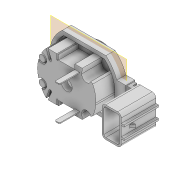
# Autodesk Inventor part: Holder750
Saved by Autodesk Inventor 2021 (Build 250183000, 183)
## iProperties
Created: 2025-07-03
Part Number: Holder750
Material: Generic
Document SubType Name: Modeling
Designer: Owner
Density: 1 g/cm^3
Appearance: Default
Author: Owner
Autodesk Inventor part; units mm, degrees
ref_plane "YZ Plane" through (0, 0, 0) normal (1, 0, 0) x (0, 1, 0)
ref_plane "XZ Plane" through (0, 0, 0) normal (0, 1, 0) x (-1, 0, 0)
ref_plane "XY Plane" through (0, 0, 0) normal (0, 0, 1) x (1, 0, 0)
sketch "Sketch1" plane through (0, 0, 0) normal (0, 0, 1) x (1, 0, 0)
  line L0 (-12, -15.2) -> (12, -15.2)
  line L1 (12, 15.2) -> (-12, 15.2)
  line L2 (-19, -15.2) -> (19, 15.2) construction
  line L3 (19, -15.2) -> (-19, 15.2) construction
  arc A0 (-12, 15.2) -> (-19, 0) centre (1.0029, 0) ccw
  arc A1 (-19, 0) -> (-12, -15.2) centre (1.0029, 0) ccw
  line L4 (-19, -15.2) -> (19, 15.2) construction
  arc A2 (19, 0) -> (12, 15.2) centre (-1.0029, 0) ccw
  arc A3 (12, -15.2) -> (19, 0) centre (-1.0029, 0) ccw
  point P0 (0, 0)
  dimension "d0" = 38
  dimension "d1" = 30.4
  dimension "d2" = 7
  constraints: 10 end point, 8 point on circle, 4 centre point, 2 midpoint, 1 horizontal, 1 parallel
  measures "d0" distance of L3.end L2.end
  measures "d1" distance of L2.end L3.start
  measures "d2" distance of L1.end L3.end
extrude "Extrusion1" add sketch "Sketch1" along normal blind 5
sketch "Sketch2" plane through (0, 0, 5) normal (0, 0, 1) x (1, 0, 0)
  arc A0 (12, -15.2) -> (12, 15.2) centre (-1.0029, 0) ccw projected
  line L0 (12, 15.2) -> (-12, 15.2) projected
  arc A1 (-12, 15.2) -> (-12, -15.2) centre (1.0029, 0) ccw projected
  line L1 (-12, -15.2) -> (12, -15.2) projected
  arc A2 (11.239, -13.2) -> (11.239, 13.2) centre (-1.0029, 0) ccw
  line L2 (11.239, -13.2) -> (-11.239, -13.2)
  arc A3 (-11.239, 13.2) -> (-11.239, -13.2) centre (1.0029, 0) ccw
  line L3 (-11.239, 13.2) -> (11.239, 13.2)
  point P0 (0, 0)
  dimension "d5" = 2
  constraints: 4 end point, 4 point on circle, 2 centre point, 3 other
  measures "d5" radial gap between concentric circles of A0 A2
extrude "Extrusion2" cut sketch "Sketch2" against normal blind 5 contours L2 A3 L3 A2
ref_plane "Work Plane1" through (0, 0, 2.5) normal (0, 0, 1) x (1, 0, 0)
sketch "Sketch3" plane through (0, 0, 2.5) normal (0, 0, 1) x (1, 0, 0)
  arc A0 (11.239, -13.2) -> (11.239, 13.2) centre (-1.0029, 0) ccw projected
  line L0 (11.239, 13.2) -> (-11.239, 13.2) projected
  arc A1 (-11.239, 13.2) -> (-11.239, -13.2) centre (1.0029, 0) ccw projected
  line L1 (-11.239, -13.2) -> (11.239, -13.2) projected
  arc A2 (12, -15.2) -> (12, 15.2) centre (-1.0029, 0) ccw projected
  line L2 (-12, -15.2) -> (12, -15.2) projected
  arc A3 (-12, 15.2) -> (-12, -15.2) centre (1.0029, 0) ccw projected
  line L3 (12, 15.2) -> (-12, 15.2) projected
  line L4 (-5.3682, -1.8242) -> (5.3682, -1.8242)
  arc A4 (5.3682, -1.8242) -> (5.3682, 1.8242) centre (-1.0029, 0) ccw
  line L5 (5.3682, 1.8242) -> (-5.3682, 1.8242)
  arc A5 (-5.3682, 1.8242) -> (-5.3682, -1.8242) centre (1.0029, 0) ccw
  point P0 (0, 0)
  constraints: 4 end point, 4 point on circle, 2 centre point, 3 other
extrude "Extrusion3" add sketch "Sketch3" against normal blind 1 contours L1 A1 L0 A0
sketch "Sketch4" plane through (0, 0, 1.5) normal (0, 0, -1) x (-1, 0, 0)
  circle A0 centre (0, 0) radius 11.25
  dimension "d10" = 22.5
  constraints: 1 centre point, 1 coincident
  measures "d10" diameter of A0
extrude "Extrusion4" add sketch "Sketch4" along normal blind 6
sketch "Sketch5" plane through (0, 0, 2.5) normal (0, 0, 1) x (1, 0, 0)
  arc A0 (11.239, -13.2) -> (11.239, 13.2) centre (-1.0029, 0) ccw projected
  line L0 (11.239, -13.2) -> (-11.239, -13.2) projected
  arc A1 (-11.239, 13.2) -> (-11.239, -13.2) centre (1.0029, 0) ccw projected
  line L1 (-11.239, 13.2) -> (11.239, 13.2) projected
  arc A2 (12, -15.2) -> (12, 15.2) centre (-1.0029, 0) ccw projected
  line L2 (12, 15.2) -> (-12, 15.2) projected
  arc A3 (-12, 15.2) -> (-12, -15.2) centre (1.0029, 0) ccw projected
  line L3 (-12, -15.2) -> (12, -15.2) projected
  arc A4 (5.3351, -1.7805) -> (5.3351, 1.7805) centre (-1.0029, 0) ccw
  line L4 (5.3351, -1.7805) -> (-5.3351, -1.7805)
  arc A5 (-5.3351, 1.7805) -> (-5.3351, -1.7805) centre (1.0029, 0) ccw
  line L5 (-5.3351, 1.7805) -> (5.3351, 1.7805)
  point P0 (0, 0)
  constraints: 4 end point, 4 point on circle, 2 centre point, 3 other
extrude "Extrusion5" add sketch "Sketch5" along normal blind 1 contours L0 A1 L1 A0
sketch "Sketch6" plane through (0, 0, 3.5) normal (0, 0, 1) x (1, 0, 0)
  arc A0 (11.239, -13.2) -> (11.239, 13.2) centre (-1.0029, 0) ccw projected
  line L0 (11.239, -13.2) -> (-11.239, -13.2) projected
  arc A1 (-11.239, 13.2) -> (-11.239, -13.2) centre (1.0029, 0) ccw projected
  line L1 (-11.239, 13.2) -> (11.239, 13.2) projected
  arc A2 (12, -15.2) -> (12, 15.2) centre (-1.0029, 0) ccw projected
  line L2 (12, 15.2) -> (-12, 15.2) projected
  arc A3 (-12, 15.2) -> (-12, -15.2) centre (1.0029, 0) ccw projected
  line L3 (-12, -15.2) -> (12, -15.2) projected
  line L4 (4.5, -14.8235) -> (-4.5, -14.8235)
  line L5 (-4.5, -9.5765) -> (4.5, -9.5765)
  line L6 (4.5, -9.5765) -> (4.5, -12.2)
  line L7 (4.5, -14.8235) -> (-4.5, -9.5765) construction
  line L8 (-4.5, -14.8235) -> (4.5, -9.5765) construction
  line L9 (-4.5, -12.2) -> (-4.5, -9.5765)
  line L10 (4.5, -12.2) -> (8.5, -12.2)
  circle A4 centre (0, 0) radius 3
  line L11 (4.5, -12.2) -> (8.5, -12.2)
  line L12 (15.9256, -1.5884) -> (15.991, -0.5538)
  arc A5 (11.239, -13.2) -> (11.239, 13.2) centre (-1.0029, 0) ccw projected
  arc A6 (13.2862, -8.3182) -> (8.2507, -9.4329) centre (10.8402, -9.1996) ccw
  arc A7 (14.2307, -7.5522) -> (14.2307, 7.5522) centre (-1.0029, 0) ccw
  line L13 (14.2307, -7.5522) -> (13.2862, -8.3182)
  line L14 (8.5, -12.2) -> (8.2507, -9.4329)
  line L15 (-4.8613, -12.2) -> (-4.8613, -9.2)
  line L16 (-4.8613, -9.2) -> (-5.3613, -9.2)
  line L17 (-5.3613, -9.2) -> (-5.3613, -12.2)
  line L18 (-10.2634, -12.2) -> (-5.3613, -12.2)
  line L19 (-4.8613, -12.2) -> (-4.5, -12.2)
  line L20 (-10.2634, -12.2) -> (-5.8402, -12.2) construction
  arc A8 (-8.3701, -7.8223) -> (-9.7725, -7.2951) centre (-9.0585, -7.5245) ccw
  line L21 (-8.3701, -7.8223) -> (-10.2634, -12.2)
  line L22 (-9.7725, -7.2951) -> (-11.2245, -11.8148)
  line L23 (-16, 0) -> (-15.9992, -0.1657)
  circle A9 centre (-13.4708, -5.9877) radius 1.75
  arc A10 (-13.7382, -8.4734) -> (-11.2245, -11.8148) centre (1.0029, 0) ccw
  line L24 (17, 0) -> (-17, 0)
  line L25 (-4.5, 9.5765) -> (4.5, 9.5765)
  line L26 (4.5, 9.5765) -> (4.5, 12.2)
  line L27 (4.5, 14.8235) -> (-4.5, 9.5765) construction
  line L28 (-4.5, 14.8235) -> (4.5, 9.5765) construction
  line L29 (-4.5, 12.2) -> (-4.5, 9.5765)
  line L30 (4.5, 12.2) -> (8.5, 12.2)
  line L31 (4.5, 12.2) -> (8.5, 12.2)
  arc A11 (8.2507, 9.4329) -> (13.2862, 8.3182) centre (10.8402, 9.1996) ccw
  line L32 (14.2307, 7.5522) -> (13.2862, 8.3182)
  line L33 (8.5, 12.2) -> (8.2507, 9.4329)
  line L34 (-4.8613, 12.2) -> (-4.8613, 9.2)
  line L35 (-4.8613, 9.2) -> (-5.3613, 9.2)
  line L36 (-5.3613, 9.2) -> (-5.3613, 12.2)
  line L37 (-10.2634, 12.2) -> (-5.3613, 12.2)
  line L38 (-4.8613, 12.2) -> (-4.5, 12.2)
  line L39 (-10.2634, 12.2) -> (-5.8402, 12.2) construction
  arc A12 (-9.7725, 7.2951) -> (-8.3701, 7.8223) centre (-9.0585, 7.5245) ccw
  line L40 (-8.3701, 7.8223) -> (-10.2634, 12.2)
  line L41 (-9.7725, 7.2951) -> (-11.2245, 11.8148)
  circle A13 centre (-13.4708, 5.9877) radius 1.75
  arc A14 (-11.2245, 11.8148) -> (-13.7382, 8.4734) centre (1.0029, 0) ccw
  line L42 (8.5, 12.2) -> (4.5, 12.2)
  line L43 (-4.5, 12.2) -> (-4.8613, 12.2)
  line L44 (-5.3613, 12.2) -> (-10.2634, 12.2)
  arc A15 (-11.2245, 11.8148) -> (-13.7382, 8.4734) centre (1.0029, 0) ccw
  arc A16 (-15.4161, 4.4175) -> (-15.4161, -4.4175) centre (1.0029, 0) ccw
  circle A17 centre (-13.4708, -5.9877) radius 2.5
  circle A18 centre (-13.4708, 5.9877) radius 2.5
  point P0 (-15.1194, -5.4008)
  point P1 (-14.2229, -7.5679)
  point P2 (15.9256, 1.5884)
  point P3 (-15.1194, 5.4008)
  point P4 (-14.2229, 7.5679)
  dimension "d16" = 9
  dimension "d17" = 6
  dimension "d18" = 4
  dimension "d19" = 6.2
  dimension "d20" = 5.2
  dimension "d21" = 0.5
  dimension "d24" = 1.5
  dimension "d27" = 3.5
  dimension "d28" = 5
  dimension "d29" = 5
  dimension "d32" = 3
  constraints: 82 end point, 32 point on circle, 25 symmetric about line, 14 centre point, 3 coincident, 3 parallel, 3 tangent, 2 horizontal, 1 perpendicular, 4 other
  measures "d16" distance of L5.start L5.end
  measures "d17" diameter of A4
  measures "d18" distance of L10.end L6.end
  measures "d19" distance of L13.start L12.start
  measures "d20" diameter of A6
  measures "d21" distance of L16.end L15.end
  measures "d24" diameter of A8
  measures "d27" diameter of A9
  measures "d28" diameter of A17
  measures "d29" diameter of A18
  measures "d32" distance of L16.end L17.end
extrude "Extrusion6" add sketch "Sketch6" along normal blind 11 contours L24 A4 A16 A18 A14 L41 A12 L40 L37 L36 L35 L34 L38 L29 L25 L26 L30 L33 A11 L32 A7 | A7 L12 L13 A6 L14 L10 L6 L5 L9 L19 L15 L16 L17 L18 L21 A8 L22 A10 A17 A16 L23 L24 A4 | A9 | A13
sketch "Sketch7" plane through (0, 0, 14.5) normal (0, 0, 1) x (1, 0, 0)
  line L0 (-4.5, -9.5765) -> (4.5, -9.5765) projected
  line L1 (4.5, -9.5765) -> (7, -9.5765)
  line L2 (7, -9.5765) -> (7, -9.0765)
  line L3 (7, -9.0765) -> (4.5, -9.0765)
  line L4 (4.5, -9.0765) -> (4.5, -9.5765)
  arc A0 (11.239, -13.2) -> (11.239, 13.2) centre (-1.0029, 0) ccw projected
  line L5 (4.5, 9.5765) -> (7, 9.5765)
  line L6 (7, 9.5765) -> (7, 9.0765)
  line L7 (7, 9.0765) -> (4.5, 9.0765)
  line L8 (4.5, 9.0765) -> (4.5, 9.5765)
  point P0 (0, 0)
  dimension "d33" = 2.5
  dimension "d34" = 0.5
  constraints: 16 end point, 2 parallel, 1 horizontal, 1 perpendicular
  measures "d33" distance of L3.end L2.end
  measures "d34" distance of L2.end L1.end
extrude "Extrusion7" add sketch "Sketch7" along normal blind 11
chamfer "Chamfer1" distance 0.5 angle 45 4 edges at (4.5, -9.3265, 25.5) (7, -9.3265, 25.5) (7, 9.3265, 25.5) (4.5, 9.3265, 25.5)
sketch "Sketch8" plane through (0, 0, 5) normal (0, 0, 1) x (1, 0, 0)
  arc A0 (12, -15.2) -> (12, 15.2) centre (-1.0029, 0) ccw projected
  line L0 (19, 6.5) -> (17.9144, 6.5)
  line L1 (19, -6.5) -> (17.9144, -6.5)
  line L2 (17.9144, -6.5) -> (22.9144, -6.5)
  line L3 (22.9144, -6.5) -> (22.9144, 6.5)
  line L4 (22.9144, 6.5) -> (17.9144, 6.5)
  point P0 (0, 0)
  point P1 (19, 0)
  dimension "d40" = 6.5
  dimension "d41" = 6.5
  dimension "d42" = 5
  constraints: 10 end point, 3 point on circle, 2 perpendicular, 1 horizontal, 1 parallel
  measures "d40" distance of point (19, 0) L1.start
  measures "d41" distance of point (19, 0) L0.start
  measures "d42" distance of L1.end L2.end
extrude "Extrusion8" add sketch "Sketch8" against normal blind 5
sketch "Sketch9" plane through (22.9144, -6.5, 5) normal (1, 0, 0) x (0, 0, -1)
  line L0 (0, 0) -> (0, 13) projected
  line L1 (0, 0) -> (5, 0) projected
  line L2 (5, 13) -> (5, 0) projected
  line L3 (0, 13) -> (5, 13) projected
  line L4 (4.5, 0.5) -> (0.5, 0.5)
  line L5 (0.5, 0.5) -> (0.5, 12.5)
  line L6 (0.5, 12.5) -> (4.5, 12.5)
  line L7 (4.5, 12.5) -> (4.5, 0.5)
  point P0 (5, 6.5)
  dimension "d45" = 0.5
  constraints: 8 end point, 3 other
  measures "d45" distance between parallel lines of L2 L7
extrude "Extrusion9" add sketch "Sketch9" along normal blind 1.5 contours L4 L5 L6 L7
sketch "Sketch10" plane through (0, 0, -4.5) normal (0, 0, -1) x (-1, 0, 0)
  circle A0 centre (0, 0) radius 11.25 projected
  circle A1 centre (0, 0) radius 9.25
  dimension "d48" = 2
  constraints: 1 centre point
  measures "d48" radial gap between concentric circles of A0 A1
extrude "Extrusion10" cut sketch "Sketch10" against normal blind 16 contours A1
sketch "Sketch11" plane through (24.4144, -6.5, 5) normal (1, 0, 0) x (0, 0, -1)
  line L0 (0.5, 0.5) -> (0.5, 12.5) projected
  line L1 (4.5, 12.5) -> (0.5, 12.5) projected
  line L2 (0.5, 0.5) -> (2.5, 0.5)
  line L3 (2.5, 0.5) -> (2.5, 12.5)
  line L4 (2.5, 12.5) -> (0.5, 12.5)
  line L5 (0.5, 12.5) -> (0.5, 0.5)
  point P0 (5, 6.5)
  dimension "d51" = 2
  constraints: 8 end point, 2 parallel, 1 horizontal, 1 midpoint, 1 perpendicular
  measures "d51" distance of L4.end L3.end
extrude "Extrusion11" add sketch "Sketch11" along normal blind 2
sketch "Sketch12" plane through (24.4144, -6, 2.5) normal (0, 0, -1) x (-1, 0, 0)
  line L0 (-2, 12) -> (-2, 0) projected
  line L1 (-2, 12.25) -> (-2, -0.25)
  line L2 (-4, 14.25) -> (-10.5, 14.25)
  line L3 (-12.5, 12.25) -> (-12.5, -0.25)
  line L4 (-10.5, -2.25) -> (-4, -2.25)
  arc A0 (-10.5, 14.25) -> (-12.5, 12.25) centre (-10.5, 12.25) ccw
  arc A1 (-2, 12.25) -> (-4, 14.25) centre (-4, 12.25) ccw
  arc A2 (-4, -2.25) -> (-2, -0.25) centre (-4, -0.25) ccw
  arc A3 (-12.5, -0.25) -> (-10.5, -2.25) centre (-10.5, -0.25) ccw
  point P0 (24.4144, 6)
  point P1 (-2, 14.25)
  point P2 (-2, -2.25)
  point P3 (-12.5, 14.25)
  dimension "d55" = 16.5
  dimension "d56" = 10.5
  dimension "d57" = 2
  constraints: 8 end point, 8 point on circle, 8 tangent, 6 point on line, 4 centre point, 3 equal radius, 2 perpendicular, 1 horizontal
  measures "d55" distance of point (-2, 14.25) point (-2, -2.25)
  measures "d56" distance of point (-2, 14.25) point (-12.5, 14.25)
  measures "d57" radius of A0
extrude "Extrusion12" add sketch "Sketch12" against normal blind 19
sketch "Sketch13" plane through (24.4144, -6, 21.5) normal (0, 0, 1) x (1, 0, 0)
  line L0 (2, 12.25) -> (2, -0.25) projected
  arc A0 (2, -0.25) -> (4, -2.25) centre (4, -0.25) ccw projected
  line L1 (4, -2.25) -> (10.5, -2.25) projected
  arc A1 (10.5, -2.25) -> (12.5, -0.25) centre (10.5, -0.25) ccw projected
  line L2 (12.5, -0.25) -> (12.5, 12.25) projected
  arc A2 (12.5, 12.25) -> (10.5, 14.25) centre (10.5, 12.25) ccw projected
  line L3 (10.5, 14.25) -> (4, 14.25) projected
  arc A3 (4, 14.25) -> (2, 12.25) centre (4, 12.25) ccw projected
  line L4 (3, 12.25) -> (3, -0.25)
  arc A4 (3, -0.25) -> (4, -1.25) centre (4, -0.25) ccw
  line L5 (4, -1.25) -> (10.5, -1.25)
  arc A5 (10.5, -1.25) -> (11.5, -0.25) centre (10.5, -0.25) ccw
  line L6 (11.5, -0.25) -> (11.5, 12.25)
  arc A6 (11.5, 12.25) -> (10.5, 13.25) centre (10.5, 12.25) ccw
  line L7 (10.5, 13.25) -> (4, 13.25)
  arc A7 (4, 13.25) -> (3, 12.25) centre (4, 12.25) ccw
  point P0 (-24.4144, 6)
  dimension "d0" = 38
  dimension "d1" = 30.4
  dimension "d2" = 7
  dimension "d60" = 1
  constraints: 8 end point, 8 point on circle, 4 centre point, 7 other
  measures "d60" radial gap between concentric circles of A3 A7
extrude "Extrusion13" cut sketch "Sketch13" against normal blind 17 contours A7 L7 A6 L6 A5 L5 A4 L4
sketch "Sketch14" plane through (24.4144, -6, 4.5) normal (0, 0, 1) x (1, 0, 0)
  line L0 (10.5, -1.25) -> (4, -1.25) projected
  line L1 (8.4598, -1.25) -> (9.6145, -1.25)
  line L2 (9.6145, -1.25) -> (9.6145, 4.1751)
  line L3 (9.6145, 4.1751) -> (8.4598, 4.1751)
  line L4 (8.4598, 4.1751) -> (8.4598, -1.25)
  line L5 (11.5, 12.25) -> (11.5, -0.25) projected
  line L6 (3, -0.25) -> (3, 12.25) projected
  line L7 (9.0371, 4.1751) -> (8.4598, 4.1751)
  line L8 (8.4598, 4.1751) -> (8.4598, 2.6751)
  line L9 (8.4598, 2.6751) -> (9.0371, 2.6751)
  line L10 (9.0371, 2.6751) -> (9.0371, 4.1751)
  line L11 (8.4598, 13.25) -> (9.6145, 13.25)
  line L12 (9.6145, 13.25) -> (9.6145, 7.8249)
  line L13 (9.6145, 7.8249) -> (8.4598, 7.8249)
  line L14 (8.4598, 7.8249) -> (8.4598, 13.25)
  line L15 (9.0371, 7.8249) -> (8.4598, 7.8249)
  line L16 (8.4598, 7.8249) -> (8.4598, 9.3249)
  line L17 (8.4598, 9.3249) -> (9.0371, 9.3249)
  line L18 (9.0371, 9.3249) -> (9.0371, 7.8249)
  point P0 (-24.4144, 6)
  dimension "d0" = 38
  dimension "d1" = 30.4
  dimension "d2" = 7
  dimension "d63" = 1.5
  constraints: 32 end point, 4 parallel, 3 point on line, 2 horizontal, 2 perpendicular, 1 midpoint
  measures "d63" distance of L8.end L7.end
extrude "Extrusion14" add sketch "Sketch14" along normal blind 12 contours L4 L3 L10 L9 | L17 L18 L13 L14
sketch "Sketch15" plane through (24.4144, -6, 4.5) normal (0, 0, 1) x (1, 0, 0)
  line L0 (10.5, -1.25) -> (4, -1.25)
  line L1 (8.4598, -1.25) -> (9.6145, -1.25)
  line L2 (9.6145, -1.25) -> (9.6145, 4.1751)
  line L3 (9.6145, 4.1751) -> (8.4598, 4.1751)
  line L4 (8.4598, 4.1751) -> (8.4598, -1.25)
  line L5 (11.5, 12.25) -> (11.5, -0.25)
  line L6 (3, -0.25) -> (3, 12.25)
  line L7 (9.0371, 4.1751) -> (8.4598, 4.1751)
  line L8 (8.4598, 4.1751) -> (8.4598, 2.6751)
  line L9 (8.4598, 2.6751) -> (9.0371, 2.6751)
  line L10 (9.0371, 2.6751) -> (9.0371, 4.1751)
  line L11 (8.4598, 13.25) -> (9.6145, 13.25)
  line L12 (9.6145, 13.25) -> (9.6145, 7.8249)
  line L13 (9.6145, 7.8249) -> (8.4598, 7.8249)
  line L14 (8.4598, 7.8249) -> (8.4598, 13.25)
  line L15 (9.0371, 7.8249) -> (8.4598, 7.8249)
  line L16 (8.4598, 7.8249) -> (8.4598, 9.3249)
  line L17 (8.4598, 9.3249) -> (9.0371, 9.3249)
  line L18 (9.0371, 9.3249) -> (9.0371, 7.8249)
  point P0 (-24.4144, 6)
  point P1 (-24.4144, 6)
  point P2 (9.6145, -1.25)
  dimension "d0" = 38
  dimension "d1" = 30.4
  dimension "d2" = 7
  dimension "d66" = 1.5
  constraints: 38 end point, 4 parallel, 3 point on line, 2 horizontal, 2 perpendicular, 1 midpoint
  measures "d66" distance of L8.end L7.end
extrude "Extrusion15" add sketch "Sketch15" along normal blind 2 contours L0 L4 L9 L10 L3 L2 | L11 L12 L13 L18 L17 L14
sketch "Sketch16" plane through (36.9144, -6.25, 2.5) normal (1, 0, 0) x (0, 0, -1)
  line L0 (-19, 0) -> (-19, 12.5) projected
  line L1 (2, 0.25) -> (2, 12.25) projected
  line L2 (0, 12.5) -> (0, 0) projected
  line L3 (-19, 8.9433) -> (0, 8.9433)
  line L4 (0, 8.9433) -> (0, 9.9433)
  line L5 (0, 9.9433) -> (-19, 9.9433)
  line L6 (-19, 9.9433) -> (-19, 8.9433)
  line L7 (-19, 3.5567) -> (0, 3.5567)
  line L8 (0, 3.5567) -> (0, 2.5567)
  line L9 (0, 2.5567) -> (-19, 2.5567)
  line L10 (-19, 2.5567) -> (-19, 3.5567)
  point P0 (2.5, 6.25)
  point P1 (-19, 2.5567)
  point P2 (0, 2.5567)
  point P3 (0, 3.5567)
  dimension "d69" = 1
  constraints: 16 end point, 2 parallel, 2 point on line, 1 horizontal, 1 perpendicular
  measures "d69" distance of L4.end L3.end
extrude "Extrusion16" add sketch "Sketch16" along normal blind 1.5 contours L0 L7 L2 L9 | L0 L5 L2 L3
sketch "Sketch17" plane through (36.9144, -2.6933, 2.5) normal (1, 0, 0) x (0, 0, -1)
  line L0 (-19, 8.9433) -> (-19, -3.5567) projected
  line L1 (-12.5, 1.9433) -> (-14.5, 1.9433)
  line L2 (-14.5, 1.9433) -> (-14.5, 3.4433)
  line L3 (-14.5, 3.4433) -> (-12.5, 3.4433)
  line L4 (-12.5, 3.4433) -> (-12.5, 1.9433)
  line L5 (-12.5, 1.9433) -> (-14.5, 3.4433) construction
  line L6 (-14.5, 1.9433) -> (-12.5, 3.4433) construction
  point P0 (2.5, 2.6933)
  dimension "d73" = 2
  dimension "d74" = 1.5
  constraints: 12 end point, 2 parallel, 1 horizontal, 1 perpendicular
  measures "d73" distance of L2.end L3.end
  measures "d74" distance of L1.end L2.end
extrude "Extrusion17" add sketch "Sketch17" along normal blind 1.5
sketch "Sketch18" plane through (36.9144, 0.75, 17) normal (0, 1, 0) x (1, 0, 0)
  line L0 (1.5, 0) -> (1.5, 2) projected
  line L1 (1.5, 2) -> (0, 0)
  line L2 (0, 0) -> (1.5, 0)
  line L3 (1.5, 0) -> (1.5, 2)
  point P0 (-36.9144, 17)
  constraints: 6 end point, 1 horizontal, 1 perpendicular
extrude "Extrusion18" cut sketch "Sketch18" against normal blind 1.5
body "Solid1"
